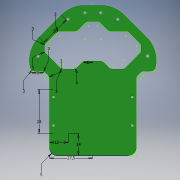
# Autodesk Inventor part: mainpcb
Saved by Autodesk Inventor 2016 (Build 200138000, 138)
## iProperties
Created: 2017-05-27
Part Number: mainpcb
Material: Ogólny
Document SubType Name: Modeling
Designer: Karol
Density: 1 g/cm^3
Appearance: Smooth - Dark Forest Green
Author: Karol
Autodesk Inventor part; units mm, degrees
ref_plane "YZ Plane" through (0, 0, 0) normal (1, 0, 0) x (0, 1, 0)
ref_plane "XZ Plane" through (0, 0, 0) normal (0, 1, 0) x (-1, 0, 0)
ref_plane "XY Plane" through (0, 0, 0) normal (0, 0, 1) x (1, 0, 0)
sketch "Sketch1" plane through (0, 0, 0) normal (0, 1, 0) x (-1, 0, 0)
  line L0 (0, 0) -> (0, 22.5)
  line L1 (5, 27.5) -> (48.7574, 27.5)
  arc A0 (5, 27.5) -> (0, 22.5) centre (5, 22.5) ccw
  arc A1 (95.1955, 5) -> (89.1353, 20) centre (73.6017, 5) ccw
  line L2 (89.1353, 20) -> (74.9931, 34.1421)
  line L3 (26, -0.0008) -> (39.959, -0.0008)
  line L4 (95.1955, 5) -> (95.1955, 0)
  line L5 (0, 0) -> (0, -22.5017)
  arc A2 (0, -22.5017) -> (5, -27.5017) centre (5, -22.5017) ccw
  line L6 (50.8787, 28.3787) -> (52.6569, 30.1569)
  line L7 (53.5355, 32.2782) -> (53.5355, 36.7771)
  arc A3 (74.9931, 34.1421) -> (55.8844, 39.7056) centre (60.372, 19.521) ccw
  line L8 (55.7045, 20.8787) -> (64.6301, 29.805)
  line L9 (66.7515, 30.6838) -> (69.1812, 30.6838)
  arc A4 (71.3027, 29.805) -> (69.1812, 30.6838) centre (69.1812, 27.6838) ccw
  arc A5 (66.7515, 30.6838) -> (64.6301, 29.805) centre (66.7515, 27.6838) ccw
  arc A6 (55.7045, 20.8787) -> (54.8259, 18.7574) centre (57.8259, 18.7574) ccw
  arc A7 (48.7574, 27.5) -> (50.8787, 28.3787) centre (48.7574, 30.5) ccw
  arc A8 (52.6569, 30.1569) -> (53.5355, 32.2782) centre (50.5355, 32.2782) ccw
  arc A9 (55.8844, 39.7056) -> (53.5355, 36.7771) centre (56.5355, 36.7771) ccw
  arc A10 (89.1353, -20.0017) -> (95.1955, -5.0017) centre (73.6017, -5.0017) ccw
  line L10 (89.1353, -20.0017) -> (74.9931, -34.1438)
  line L11 (95.1955, -5.0017) -> (95.1955, 0)
  line L12 (50.8787, -28.3804) -> (52.6569, -30.1585)
  line L13 (53.5355, -32.2799) -> (53.5355, -36.7788)
  arc A11 (55.8844, -39.7072) -> (74.9931, -34.1438) centre (60.372, -19.5227) ccw
  arc A12 (50.8787, -28.3804) -> (48.7574, -27.5017) centre (48.7574, -30.5017) ccw
  arc A13 (53.5355, -32.2799) -> (52.6569, -30.1585) centre (50.5355, -32.2799) ccw
  arc A14 (53.5355, -36.7788) -> (55.8844, -39.7072) centre (56.5355, -36.7788) ccw
  line L14 (48.7574, -27.5017) -> (5, -27.5017)
  line L15 (71.3027, 29.805) -> (78.0002, 23.1064)
  line L16 (78.8787, 20.9852) -> (78.8787, 11.3601)
  line L17 (79.7568, 9.2393) -> (84.1169, 4.8769)
  arc A15 (78.8787, 20.9852) -> (78.0002, 23.1064) centre (75.8787, 20.9852) ccw
  arc A16 (78.8787, 11.3601) -> (79.7568, 9.2393) centre (81.8787, 11.3601) ccw
  arc A17 (84.995, 2.7562) -> (84.1169, 4.8769) centre (81.995, 2.7562) ccw
  line L18 (84.995, 2.7562) -> (84.995, 0)
  line L19 (78.8787, -20.9869) -> (78.8787, -11.3618)
  line L20 (79.7568, -9.241) -> (84.1169, -4.8786)
  arc A18 (79.7568, -9.241) -> (78.8787, -11.3618) centre (81.8787, -11.3618) ccw
  arc A19 (84.1169, -4.8786) -> (84.995, -2.7578) centre (81.995, -2.7578) ccw
  line L21 (84.995, 0) -> (84.995, -2.7578)
  line L22 (55.7045, -20.8804) -> (64.6301, -29.8067)
  line L23 (66.7515, -30.6855) -> (69.1812, -30.6855)
  arc A20 (69.1812, -30.6855) -> (71.3027, -29.8066) centre (69.1812, -27.6855) ccw
  arc A21 (64.6301, -29.8067) -> (66.7515, -30.6855) centre (66.7515, -27.6855) ccw
  arc A22 (54.8259, -18.7591) -> (55.7045, -20.8804) centre (57.8259, -18.7591) ccw
  line L24 (71.3027, -29.8066) -> (78.0002, -23.1081)
  arc A23 (78.0002, -23.1081) -> (78.8787, -20.9869) centre (75.8787, -20.9869) ccw
  line L25 (59.826, 0) -> (59.826, 4.7574)
  line L26 (58.9473, 6.8787) -> (55.7046, 10.1214)
  line L27 (54.8259, 18.7574) -> (54.8259, 12.2428)
  arc A24 (54.8259, 12.2428) -> (55.7046, 10.1214) centre (57.8259, 12.2428) ccw
  arc A25 (59.826, 4.7574) -> (58.9473, 6.8787) centre (56.826, 4.7574) ccw
  line L28 (58.9473, -6.8804) -> (55.7046, -10.1231)
  arc A26 (55.7046, -10.1231) -> (54.8259, -12.2445) centre (57.8259, -12.2445) ccw
  arc A27 (58.9473, -6.8804) -> (59.826, -4.7591) centre (56.826, -4.7591) ccw
  line L29 (54.8259, -12.2445) -> (54.8259, -18.7591)
  line L30 (59.826, 0) -> (59.826, -4.7591)
  point P0 (0, 27.5)
  point P1 (42, 25)
  point P2 (14, 25)
  point P3 (14, 15.5)
  point P4 (37, 24.9983)
  point P5 (19, 24.9983)
  point P6 (0, -27.5017)
  point P7 (42, -25.0017)
  point P8 (14, -25.0017)
  point P9 (14, -15.5017)
  point P10 (37, -25)
  point P11 (19, -25)
  point P12 (53.5355, 31.0355)
  point P13 (53.5355, 39.0355)
  point P14 (70.4238, 30.6838)
  point P15 (54.8259, 20)
  point P16 (65.5088, 30.6838)
  point P17 (53.5355, -31.0372)
  point P18 (53.5355, -39.0372)
  point P19 (84.995, 3.9983)
  point P20 (84.995, -4)
  point P21 (60.372, -19.5227)
  point P22 (70.4238, -30.6855)
  point P23 (54.8259, -20.0017)
  point P24 (59.826, 6)
  point P25 (59.826, -6.0017)
  point P26 (63.036, 34.776)
  point P27 (86.3487, 15.8276)
  point P28 (90.4692, 5.0078)
  point P29 (63.036, -34.7777)
  point P30 (86.3487, -15.8293)
  point P31 (90.4692, -5.0095)
  dimension "d2" = 27.5
  dimension "d19" = 5
  dimension "d43" = 28
  dimension "d45" = 12
  dimension "d73" = 20
  dimension "d118" = 8
  dimension "d124" = 3
  dimension "d125" = 3
  dimension "d126" = 3
  dimension "d127" = 3
  dimension "d128" = 3
  dimension "d129" = 3
  dimension "d133" = 14
  dimension "d147" = 3
  dimension "d148" = 6
  dimension "d149" = 3
  constraints: 62 end point, 59 symmetric about line, 58 point on circle, 28 centre point, 23 tangent, 20 point on line, 10 vertical, 4 horizontal, 3 equal radius, 14 other
  measures "d2" distance of L0.start point (0, 27.5)
  measures "d19" radius of A0
  measures "d43" distance of point (14, 25) point (42, 25)
  measures "d45" distance from line of L1 point (14, 15.5)
  measures "d73" distance of L2.start L2.end
  measures "d118" distance of point (53.536, 31.036) point (53.536, 39.036)
  measures "d124" radius of A4
  measures "d125" radius of A5
  measures "d126" radius of A6
  measures "d127" radius of A7
  measures "d128" radius of A8
  measures "d129" radius of A9
  measures "d133" distance from line of L0 point (14, 15.5)
  measures "d147" radius of A15
  measures "d148" distance of L25.start point (59.826, 6)
  measures "d149" radius of A24
extrude "Extrusion1" add sketch "Sketch1" along normal blind 1.4
hole "Hole1" at (-37, 0, 24.9983) at (-19, 0, 24.9983) at (-37, 0, -25) at (-19, 0, -25) direction (0, 1, 0) diameter 2 depth 2 tip angle 118
hole "Hole3" at (-14, 0, 15.5) direction (0, 1, 0) diameter 0.1 depth 8 tip angle 118
hole "Hole5" at (-63.036, 0, 34.776) at (-86.3487, 0, 15.8276) at (-90.4692, 0, 5.0078) at (-63.036, 0, -34.7777) at (-86.3487, 0, -15.8293) at (-90.4692, 0, -5.0095) direction (0, 1, 0) diameter 2.5 depth 8 tip angle 118
body "Solid1"
